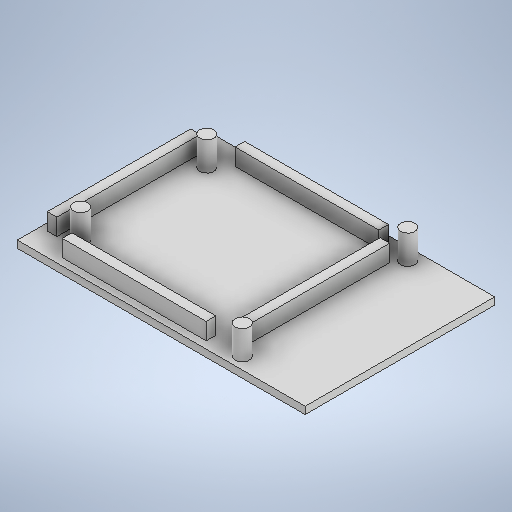
# Autodesk Inventor part: RFID-RC522 Holder 3.3
Saved by Autodesk Inventor 2025.2 (Build 292293000, 293)
## iProperties
Created: 2024-11-16
Part Number: RFID-RC522 Holder 3.3
Material: Generic
Document SubType Name: Modeling
Designer: jurre
Density: 1 g/cm^3
Appearance: Default
Author: jurre
Autodesk Inventor part; units mm, degrees
ref_plane "YZ Plane" through (0, 0, 0) normal (1, 0, 0) x (0, 1, 0)
ref_plane "XZ Plane" through (0, 0, 0) normal (0, 1, 0) x (-1, 0, 0)
ref_plane "XY Plane" through (0, 0, 0) normal (0, 0, 1) x (1, 0, 0)
sketch "Sketch5" plane through (0, 0, 0) normal (0, 1, 0) x (-1, 0, 0)
  line L0 (9.5203, 12.3105) -> (-50.4797, 12.3105)
  line L1 (-50.4797, 12.3105) -> (-50.4797, -27.1895)
  line L2 (-50.4797, -27.1895) -> (9.5203, -27.1895)
  line L3 (9.5203, -27.1895) -> (9.5203, 12.3105)
  line L4 (-33.3579, -22.4395) -> (-31.3579, -22.4395)
  line L5 (-31.3579, -22.4395) -> (-31.3579, 7.5605)
  line L6 (-31.3579, 7.5605) -> (-33.3579, 7.5605)
  line L7 (-33.3579, 7.5605) -> (-33.3579, -22.4395)
  line L8 (8.0203, 7.5605) -> (6.0203, 7.5605)
  line L9 (6.0203, 7.5605) -> (6.0203, -22.3395)
  line L10 (6.0203, -22.3395) -> (8.0203, -22.3395)
  line L11 (8.0203, -22.3395) -> (8.0203, 7.5605)
  circle A0 centre (2.9203, -20.5895) radius 1.5
  circle A1 centre (2.9203, 5.7105) radius 1.5
  circle A2 centre (-34.8579, -24.6895) radius 1.5
  circle A3 centre (-34.8579, 9.8105) radius 1.5
  line L12 (-28.3579, 10.8105) -> (1.6421, 10.8105)
  line L13 (1.6421, 10.8105) -> (1.6421, 8.8105)
  line L14 (1.6421, 8.8105) -> (-28.3579, 8.8105)
  line L15 (-28.3579, 8.8105) -> (-28.3579, 10.8105)
  line L16 (-29.8579, -23.6895) -> (0.1421, -23.6895)
  line L17 (0.1421, -23.6895) -> (0.1421, -25.6895)
  line L18 (0.1421, -25.6895) -> (-29.8579, -25.6895)
  line L19 (-29.8579, -25.6895) -> (-29.8579, -23.6895)
  point P0 (0, 0)
  point P1 (-29.8579, -24.6895)
  dimension "d9" = 60
  dimension "d10" = 39.5
  dimension "d24" = 2
  dimension "d27" = 4.75
  dimension "d29" = 2
  dimension "d31" = 1.5
  dimension "d32" = 4.75
  dimension "d33" = 4.85
  dimension "d40" = 3
  dimension "d41" = 6.6
  dimension "d42" = 6.6
  dimension "d43" = 3
  dimension "d44" = 6.6
  dimension "d45" = 6.6
  dimension "d46" = 3
  dimension "d47" = 2.5
  dimension "d49" = 3
  dimension "d50" = 2.5
  dimension "d59" = 35
  dimension "d62" = 1.5
  dimension "d66" = 35
  dimension "d73" = 1.5
  dimension "d74" = 30
  dimension "d75" = 5
  dimension "d76" = 2
  dimension "d77" = 5
  dimension "d78" = 1.5
  dimension "d79" = 30
  dimension "d80" = 2
  constraints: 40 end point, 10 parallel, 5 horizontal, 5 perpendicular, 4 centre point, 1 midpoint
  measures "d9" distance of L2.end L1.end
  measures "d10" distance of L1.end L0.end
  measures "d24" distance of L6.end L5.end
  measures "d27" distance between parallel lines of L0 L6
  measures "d29" distance of L10.end L9.end
  measures "d31" distance between parallel lines of L3 L11
  measures "d32" distance between parallel lines of L0 L8
  measures "d33" distance between parallel lines of L2 L10
  measures "d40" diameter of A0
  measures "d41" distance from line of L2 A0.centre
  measures "d42" distance from line of L3 A0.centre
  measures "d43" diameter of A1
  measures "d44" distance from line of L0 A1.centre
  measures "d45" distance from line of L3 A1.centre
  measures "d46" diameter of A2
  measures "d47" distance from line of L2 A2.centre
  measures "d49" diameter of A3
  measures "d50" distance from line of L0 A3.centre
  measures "d62" distance from line of L7 A2.centre
  measures "d73" distance between parallel lines of L2 L18
  measures "d74" distance of L16.start L16.end
  measures "d75" distance of A2.centre point (-29.858, -24.689)
  measures "d76" distance of L16.end L17.end
  measures "d77" distance edge to line of A3 L15
  measures "d78" distance between parallel lines of L0 L12
  measures "d79" distance of L13.end L14.end
  measures "d80" distance of L12.end L13.end
extrude "Extrusion8" add sketch "Sketch5" against normal blind 1.5 contours L3 L2 L1 L0 | L7 L6 L5 L4 | L11 L10 L9 L8 | A0 | A1 | A2 | A3 | L12 L13 L14 L15 | L16 L17 L18 L19
extrude "Extrusion9" add sketch "Sketch5" along normal blind 3.5 contours L7 L6 L5 L4 | L11 L10 L9 L8 | L12 L13 L14 L15 | L16 L17 L18 L19
extrude "Extrusion10" add sketch "Sketch5" along normal blind 6 contours A0 | A1 | A2 | A3
body "Solid4"
